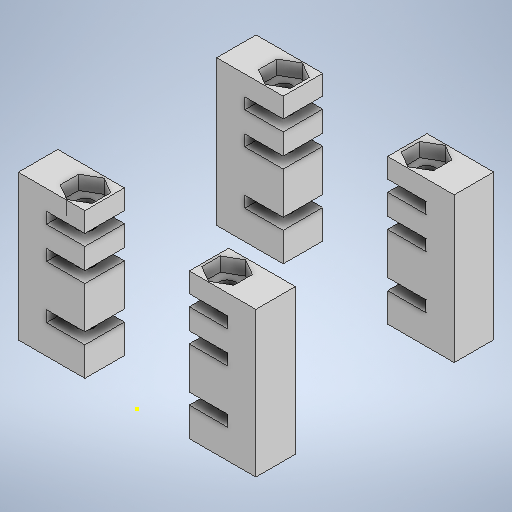
# Autodesk Inventor part: Spacer for PCB boards
Saved by Autodesk Inventor 2025 (Build 290162000, 162)
## iProperties
Created: 2024-07-10
Part Number: Spacer for PCB boards
Material: Generic
Document SubType Name: Modeling
Designer: track
Density: 1 g/cm^3
Appearance: Default
Author: track
## iProperties of the stored document Spacer for PCB boards_3DPrint.ipt
Created: 2024-07-10
Part Number: Spacer for PCB boards_3DPrint
Material: Generic
Document SubType Name: Modeling
Designer: track
Density: 1 g/cm^3
Appearance: Default
Author: track
Autodesk Inventor part; units mm, degrees
ref_plane "YZ Plane" through (0, 0, 0) normal (1, 0, 0) x (0, 1, 0)
ref_plane "XZ Plane" through (0, 0, 0) normal (0, 1, 0) x (-1, 0, 0)
ref_plane "XY Plane" through (0, 0, 0) normal (0, 0, 1) x (1, 0, 0)
sketch "Sketch8" plane through (0, 0, 0) normal (0, 1, 0) x (-1, 0, 0)
  line L0 (-16.05, 21.075) -> (16.05, 21.075)
  line L1 (16.05, 21.075) -> (16.05, -21.075)
  line L2 (16.05, -21.075) -> (-16.05, -21.075)
  line L3 (-16.05, -21.075) -> (-16.05, 21.075)
  line L4 (-16.05, 21.075) -> (16.05, -21.075) construction
  line L5 (16.05, 21.075) -> (-16.05, -21.075) construction
  circle A0 centre (12.65, -17.575) radius 1.5
  line L6 (12.65, -19.075) -> (12.65, -21.075) construction
  line L7 (14.15, -17.575) -> (16.05, -17.575) construction
  line L8 (12.65, -17.575) -> (12.65, -19.075) construction
  line L9 (12.65, -17.575) -> (14.15, -17.575) construction
  line L10 (0, -21.075) -> (0, 21.075) construction
  line L11 (16.05, 0) -> (-16.05, 0) construction
  line L12 (9.25, -14.075) -> (16.05, -14.075)
  line L13 (16.05, -14.075) -> (16.05, -21.075)
  line L14 (16.05, -21.075) -> (9.25, -21.075)
  line L15 (9.25, -21.075) -> (9.25, -14.075)
  line L16 (9.25, -14.075) -> (16.05, -21.075) construction
  line L17 (16.05, -14.075) -> (9.25, -21.075) construction
  circle A1 centre (-12.55, -17.675) radius 1.5
  line L18 (-9.25, -14.075) -> (-16.05, -14.075)
  line L19 (-9.25, -21.075) -> (-9.25, -14.075)
  circle A2 centre (12.55, 17.675) radius 1.5
  line L20 (9.25, 14.075) -> (16.05, 14.075)
  line L21 (9.25, 21.075) -> (9.25, 14.075)
  line L22 (-9.25, 21.075) -> (-9.25, 14.075)
  circle A3 centre (-12.55, 17.475) radius 1.5
  line L23 (-9.25, 14.075) -> (-16.05, 14.075)
  line L24 (16.05, -21.075) -> (22.85, -21.075)
  line L25 (22.85, -21.075) -> (22.85, -14.075)
  line L26 (22.85, -14.075) -> (16.05, -14.075)
  line L27 (16.05, -14.075) -> (16.05, -21.075)
  line L28 (-16.05, -21.075) -> (-22.85, -21.075)
  line L29 (-22.85, -21.075) -> (-22.85, -14.075)
  line L30 (-22.85, -14.075) -> (-16.05, -14.075)
  line L31 (16.05, 21.075) -> (22.85, 21.075)
  line L32 (22.85, 21.075) -> (22.85, 14.075)
  line L33 (22.85, 14.075) -> (16.05, 14.075)
  line L34 (-16.05, 21.075) -> (-22.85, 21.075)
  line L35 (-22.85, 21.075) -> (-22.85, 14.075)
  line L36 (-22.85, 14.075) -> (-16.05, 14.075)
  line L37 (-12.55, -19.175) -> (-12.55, -21.075) construction
  line L38 (-14.05, -17.675) -> (-16.05, -17.675) construction
  line L39 (-14.05, -17.675) -> (-12.55, -17.675) construction
  line L40 (-12.55, -17.675) -> (-12.55, -19.175) construction
  line L41 (-12.55, 17.475) -> (-12.55, 18.975) construction
  line L42 (-12.55, 21.075) -> (-12.55, 18.975) construction
  line L43 (-12.55, 17.475) -> (-14.05, 17.475) construction
  line L44 (-16.05, 17.475) -> (-14.05, 17.475) construction
  line L45 (12.55, 17.675) -> (12.55, 19.175) construction
  line L46 (12.55, 19.175) -> (12.55, 21.075) construction
  line L47 (12.55, 17.675) -> (14.05, 17.675) construction
  line L48 (16.05, 17.675) -> (14.05, 17.675) construction
  point P0 (0, 0)
  dimension "d65" = 42.15
  dimension "d66" = 32.1
  dimension "d67" = 3
  dimension "d69" = 2
  dimension "d70" = 1.9
  dimension "d113" = 3
  dimension "d115" = 1.9
  dimension "d116" = 2
  dimension "d117" = 2
  dimension "d118" = 2.1
  dimension "d119" = 3
  dimension "d120" = 1.9
  dimension "d121" = 2
  dimension "d122" = 3
  constraints: 98 end point, 18 symmetric about line, 11 perpendicular, 10 point on line, 9 point on circle, 8 midpoint, 6 horizontal, 6 parallel, 4 centre point, 3 collinear, 2 equal length, 2 vertical
  measures "d65" distance of L2.end L0.start
  measures "d66" distance of L1.end L2.end
  measures "d67" diameter of A0
  measures "d69" distance of L6.start L6.end
  measures "d70" distance of L7.start L7.end
  measures "d113" diameter of A1
  measures "d115" distance of L37.start L37.end
  measures "d116" distance of L38.start L38.end
  measures "d117" distance of L44.start L43.end
  measures "d118" distance of L42.start L41.end
  measures "d119" diameter of A3
  measures "d120" distance of L45.end L46.end
  measures "d121" distance of L48.start L47.end
  measures "d122" diameter of A2
extrude "Extrusion4" add sketch "Sketch8" along normal blind 1 contours L0 L22 L23 L3 | L3 L36 L35 L34 | L0 L1 L20 L21 | L18 L19 L2 L3 | L3 L28 L29 L30 | L31 L32 L33 L1 | L26 L25 L24 L1 | L1 L2 L15 L12
sketch "Sketch9" plane through (0, 1, 0) normal (0, 1, 0) x (1, 0, 0)
  line L0 (-22.85, 21.075) -> (-22.85, 14.075) projected
  line L1 (-22.85, 21.075) -> (-16.05, 21.075)
  line L2 (-16.05, 21.075) -> (-16.05, 14.075)
  line L3 (-16.05, 14.075) -> (-22.85, 14.075)
  line L4 (-22.85, 14.075) -> (-22.85, 21.075)
  line L5 (-9.25, 21.075) -> (-22.85, 21.075) projected
  line L6 (-16.05, 21.075) -> (-16.05, 14.075) construction
  line L7 (-22.85, 14.075) -> (-9.25, 14.075) projected
  line L8 (0, 20.6342) -> (0, -21.4805) construction
  line L9 (-22.8069, 0) -> (21.3685, 0) construction
  line L10 (22.85, 21.075) -> (22.85, 14.075)
  line L11 (22.85, 21.075) -> (16.05, 21.075)
  line L12 (16.05, 21.075) -> (16.05, 14.075)
  line L13 (16.05, 14.075) -> (22.85, 14.075)
  line L14 (22.85, 14.075) -> (22.85, 21.075)
  line L15 (16.05, 21.075) -> (22.85, 21.075)
  line L16 (22.85, 14.075) -> (16.05, 14.075)
  line L17 (-22.85, -21.075) -> (-22.85, -14.075)
  line L18 (-22.85, -21.075) -> (-16.05, -21.075)
  line L19 (-16.05, -21.075) -> (-16.05, -14.075)
  line L20 (-16.05, -14.075) -> (-22.85, -14.075)
  line L21 (-22.85, -14.075) -> (-22.85, -21.075)
  line L22 (-16.05, -21.075) -> (-22.85, -21.075)
  line L23 (-16.05, -21.075) -> (-16.05, -14.075) construction
  line L24 (-22.85, -14.075) -> (-16.05, -14.075)
  line L25 (0, -20.6342) -> (0, 21.4805) construction
  line L26 (22.85, -21.075) -> (22.85, -14.075)
  line L27 (22.85, -21.075) -> (16.05, -21.075)
  line L28 (16.05, -14.075) -> (22.85, -14.075)
  line L29 (22.85, -14.075) -> (22.85, -21.075)
  line L30 (16.05, -21.075) -> (22.85, -21.075)
  line L31 (22.85, -14.075) -> (16.05, -14.075)
  line L32 (16.05, -21.075) -> (16.05, -14.075)
  point P0 (0, 0)
  point P1 (9.25, 21.075)
  point P2 (9.25, 14.075)
  point P3 (-9.25, -21.075)
  point P4 (-9.25, -14.075)
  point P5 (9.25, -21.075)
  point P6 (9.25, -14.075)
  dimension "d73" = 0
  dimension "d74" = 0
  constraints: 60 end point, 25 symmetric about line, 2 collinear, 2 horizontal, 2 midpoint, 2 parallel, 1 vertical
  measures "d73" distance from line of point (0, 0) L8
  measures "d74" distance from line of point (0, 0) L9
extrude "Extrusion5" add sketch "Sketch9" along normal blind 22.241
sketch "Sketch11" plane through (-16.05, 1, 21.075) normal (1, 0, 0) x (0, 0, -1)
  line L0 (21.075, -1) -> (21.075, 11.5) construction
  line L1 (0, 0) -> (0, 22.241) projected
  line L2 (7, 0) -> (7, 22.241) projected
  line L3 (0, 4.15) -> (7, 4.15)
  line L4 (0, -1) -> (7, -1) projected
  line L5 (0, 6.15) -> (7, 6.15)
  line L6 (7, -1) -> (7, 22.241) projected
  line L7 (0, 3.15) -> (7, 3.15)
  line L8 (0, 7.15) -> (7, 7.15)
  line L9 (0, 12.55) -> (7, 12.55)
  line L10 (0, 13.55) -> (7, 13.55)
  line L11 (0, 15.55) -> (7, 15.55)
  line L12 (0, 0) -> (0, 22.3006)
  line L13 (7, 0) -> (7, 22.3006)
  line L14 (0, 16.55) -> (7, 16.55)
  line L15 (0, 19.25) -> (7, 19.25)
  line L16 (0, 18.25) -> (7, 18.25)
  line L17 (0, 21.25) -> (7, 21.25)
  line L18 (0, 22.25) -> (7, 22.25)
  line L19 (42.15, 0) -> (42.15, 22.241)
  line L20 (35.15, 0) -> (35.15, 22.241)
  line L21 (42.15, 4.15) -> (35.15, 4.15)
  line L22 (42.15, 6.15) -> (35.15, 6.15)
  line L23 (35.15, -1) -> (35.15, 22.241)
  line L24 (42.15, 3.15) -> (35.15, 3.15)
  line L25 (42.15, 7.15) -> (35.15, 7.15)
  line L26 (42.15, 12.55) -> (35.15, 12.55)
  line L27 (42.15, 13.55) -> (35.15, 13.55)
  line L28 (42.15, 15.55) -> (35.15, 15.55)
  line L29 (42.15, 0) -> (42.15, 22.3006)
  line L30 (35.15, 0) -> (35.15, 22.3006)
  line L31 (42.15, 16.55) -> (35.15, 16.55)
  line L32 (42.15, 19.25) -> (35.15, 19.25)
  line L33 (42.15, 18.25) -> (35.15, 18.25)
  line L34 (42.15, 21.25) -> (35.15, 21.25)
  line L35 (42.15, 22.25) -> (35.15, 22.25)
  line L36 (0, 0) -> (7, 0)
  line L37 (35.15, 0) -> (42.15, 0)
  point P0 (7, 15.55)
  point P1 (7, 22.241)
  point P2 (7, 13.55)
  point P3 (7, 7.15)
  point P4 (7, 6.15)
  point P5 (7, 3.15)
  point P6 (42.15, 7.15)
  point P7 (35.15, 7.15)
  point P8 (35.15, 6.15)
  point P9 (0, 15.55)
  point P10 (7, 15.55)
  point P11 (7, 18.25)
  point P12 (0, 18.25)
  point P13 (7, 16.55)
  dimension "d97" = 5.15
  dimension "d98" = 1
  dimension "d99" = 2
  dimension "d100" = 1
  dimension "d101" = 8.4
  dimension "d102" = 1
  dimension "d103" = 2
  dimension "d104" = 1
  dimension "d105" = 2.7
  dimension "d106" = 1
  dimension "d107" = 1
  dimension "d108" = 2
  constraints: 64 end point, 31 symmetric about line, 24 point on line, 11 perpendicular, 2 horizontal, 2 vertical, 1 collinear, 34 other
  measures "d97" distance between parallel lines of L4 L3
  measures "d98" distance between parallel lines of L3 L7
  measures "d99" distance between parallel lines of L3 L5
  measures "d100" distance between parallel lines of L5 L8
  measures "d101" distance between parallel lines of L9 L3
  measures "d102" distance between parallel lines of L9 L10
  measures "d103" distance between parallel lines of L10 L11
  measures "d104" distance between parallel lines of L14 L11
  measures "d105" distance between parallel lines of L15 L14
  measures "d106" distance between parallel lines of L15 L16
  measures "d107" distance between parallel lines of L17 L18
  measures "d108" distance between parallel lines of L15 L17
extrude "Extrusion6" add sketch "Sketch11" along normal up to surface (6.8 mm away) contours L1 L7 L2 L36 | L1 L3 L2 L7 | L1 L8 L2 L5 | L1 L9 L2 L8 | L1 L10 L2 L9 | L1 L14 L2 L11 | L1 L16 L2 L14 | L1 L15 L2 L16 | L1 L12 L18 L13 L2 L17 | L37 L20 L24 L19 | L24 L20 L21 L19 | L22 L20 L25 L19 | L25 L20 L26 L19 | L26 L20 L27 L19 | L28 L20 L31 L19 | L31 L20 L33 L19 | L33 L20 L32 L19 | L34 L20 L30 L35 L29 L19
sketch "Sketch12" plane through (16.05, 1, 14.075) normal (-1, 0, 0) x (0, 0, 1)
  line L0 (7, -1) -> (0, -1) projected
  line L1 (0, -1) -> (0, 4.15) projected
  line L2 (7, 4.15) -> (0, 4.15) projected
  line L3 (7, -1) -> (7, 4.15) projected
  line L4 (7, 13.55) -> (0, 13.55) projected
  line L5 (7, 6.15) -> (7, 13.55) projected
  line L6 (0, 6.15) -> (7, 6.15) projected
  line L7 (0, 13.55) -> (0, 6.15) projected
  line L8 (0, 15.55) -> (7, 15.55) projected
  line L9 (0, 19.25) -> (0, 15.55) projected
  line L10 (7, 19.25) -> (0, 19.25) projected
  line L11 (7, 15.55) -> (7, 19.25) projected
  line L12 (7, 22.25) -> (0, 22.25) projected
  line L13 (7, 21.25) -> (7, 22.25) projected
  line L14 (0, 21.25) -> (7, 21.25) projected
  line L15 (0, 22.25) -> (0, 21.25) projected
  line L16 (-28.15, 21.25) -> (-28.15, 22.25) projected
  line L17 (-35.15, 21.25) -> (-28.15, 21.25) projected
  line L18 (-35.15, 22.25) -> (-35.15, 21.25) projected
  line L19 (-28.15, 22.25) -> (-35.15, 22.25) projected
  line L20 (-35.15, 15.55) -> (-28.15, 15.55) projected
  line L21 (-28.15, 15.55) -> (-28.15, 19.25) projected
  line L22 (-35.15, 15.55) -> (-28.15, 15.55) projected
  line L23 (-35.15, 19.25) -> (-35.15, 15.55) projected
  line L24 (-28.15, 19.25) -> (-35.15, 19.25) projected
  line L25 (-35.15, 6.15) -> (-28.15, 6.15) projected
  line L26 (-35.15, 13.55) -> (-35.15, 6.15) projected
  line L27 (-28.15, 13.55) -> (-35.15, 13.55) projected
  line L28 (-28.15, 6.15) -> (-28.15, 13.55) projected
  line L29 (-28.15, -1) -> (-35.15, -1) projected
  line L30 (-35.15, -1) -> (-35.15, 4.15) projected
  line L31 (-28.15, 4.15) -> (-35.15, 4.15) projected
  line L32 (-28.15, -1) -> (-28.15, 4.15) projected
extrude "Extrusion7" add sketch "Sketch12" along normal up to surface (6.8 mm away)
sketch "Sketch13" plane through (0, 0, 0) normal (0, -1, 0) x (1, 0, 0)
  line L0 (-22.85, -14.075) -> (-16.05, -14.075) projected
  line L1 (-22.85, -14.075) -> (-21.05, -14.075)
  line L2 (-21.05, -14.075) -> (-21.05, -21.075)
  line L3 (-21.05, -21.075) -> (-22.85, -21.075)
  line L4 (-22.85, -21.075) -> (-22.85, -14.075)
  line L5 (0, 0) -> (0, -21.075) construction
  line L6 (0, 0) -> (23.0249, 0) construction
  line L7 (22.85, -14.075) -> (9.25, -14.075)
  line L8 (22.85, -21.075) -> (9.25, -21.075)
  line L9 (22.85, -14.075) -> (21.05, -14.075)
  line L10 (21.05, -14.075) -> (21.05, -21.075)
  line L11 (21.05, -21.075) -> (22.85, -21.075)
  line L12 (22.85, -21.075) -> (22.85, -14.075)
  line L13 (-22.85, 14.075) -> (-9.25, 14.075)
  line L14 (-22.85, 21.075) -> (-9.25, 21.075)
  line L15 (-22.85, 14.075) -> (-21.05, 14.075)
  line L16 (-21.05, 14.075) -> (-21.05, 21.075)
  line L17 (-21.05, 21.075) -> (-22.85, 21.075)
  line L18 (-22.85, 21.075) -> (-22.85, 14.075)
  line L19 (-16.05, 21.075) -> (-16.05, 14.075)
  line L20 (0, 0) -> (0, 21.075) construction
  line L21 (22.85, 14.075) -> (9.25, 14.075)
  line L22 (22.85, 21.075) -> (9.25, 21.075)
  line L23 (22.85, 14.075) -> (21.05, 14.075)
  line L24 (21.05, 14.075) -> (21.05, 21.075)
  line L25 (21.05, 21.075) -> (22.85, 21.075)
  line L26 (22.85, 21.075) -> (22.85, 14.075)
  circle A0 centre (-12.65, -17.575) radius 1.5
  circle A1 centre (-12.65, -17.575) radius 1.5 projected
  line L27 (-16.05, -14.075) -> (-9.25, -14.075) projected
  line L28 (-16.05, -21.075) -> (-16.05, -14.075) projected
  line L29 (-16.05, -14.075) -> (-16.05, -21.075)
  circle A2 centre (-12.55, 17.675) radius 1.5
  circle A3 centre (-12.55, 17.675) radius 1.5 projected
  circle A4 centre (12.65, -17.575) radius 1.5
  circle A5 centre (12.55, 17.675) radius 1.5
  line L30 (-22.85, -14.075) -> (-9.25, -14.075) projected
  line L31 (-9.25, -21.075) -> (-22.85, -21.075) projected
  point P0 (-21.05, 14.075)
  point P1 (21.05, 14.075)
  point P2 (21.05, -14.075)
  dimension "d109" = 5
  dimension "d111" = 3
  constraints: 54 end point, 26 symmetric about line, 4 centre point, 4 concentric, 3 coincident, 3 equal length, 3 point on line, 2 horizontal, 2 midpoint, 1 perpendicular, 1 vertical, 2 other
  measures "d109" distance between parallel lines of L2 L28
  measures "d111" diameter of A2
extrude "Extrusion8" cut sketch "Sketch13" against normal through all contours L0 L2 L3 L4 | L12 L8 L10 L7 | L18 L14 L16 L13 | L21 L24 L22 L26 | A0 | A2 | A4 | A5
sketch "Sketch14" plane through (0, 23.241, 0) normal (0, 1, 0) x (1, 0, 0)
  circle A0 centre (12.55, -17.675) radius 1.5 projected
  line L0 (9.7, -16.0296) -> (12.55, -14.3841)
  line L1 (12.55, -14.3841) -> (15.4, -16.0296)
  line L2 (15.4, -16.0296) -> (15.4, -19.3204)
  line L3 (15.4, -19.3204) -> (12.55, -20.9659)
  line L4 (12.55, -20.9659) -> (9.7, -19.3204)
  line L5 (9.7, -19.3204) -> (9.7, -16.0296)
  line L6 (0, 0) -> (0, 9.6595)
  line L7 (0, 9.6595) -> (0, 0)
  line L8 (0, 0) -> (7.0736, 0)
  circle A1 centre (12.55, -17.675) radius 1.5
  circle A2 centre (12.65, 17.575) radius 1.5 projected
  line L9 (9.8, 19.2204) -> (12.65, 20.8659)
  line L10 (12.65, 20.8659) -> (15.5, 19.2204)
  line L11 (15.5, 19.2204) -> (15.5, 15.9296)
  line L12 (15.5, 15.9296) -> (12.65, 14.2841)
  line L13 (12.65, 14.2841) -> (9.8, 15.9296)
  line L14 (9.8, 15.9296) -> (9.8, 19.2204)
  circle A3 centre (-12.55, -17.675) radius 1.5 projected
  line L15 (-15.4, -16.0296) -> (-12.55, -14.3841)
  line L16 (-12.55, -14.3841) -> (-9.7, -16.0296)
  line L17 (-9.7, -16.0296) -> (-9.7, -19.3204)
  line L18 (-9.7, -19.3204) -> (-12.55, -20.9659)
  line L19 (-12.55, -20.9659) -> (-15.4, -19.3204)
  line L20 (-15.4, -19.3204) -> (-15.4, -16.0296)
  circle A4 centre (-12.65, 17.575) radius 1.5 projected
  line L21 (-15.5, 19.2204) -> (-12.65, 20.8659)
  line L22 (-12.65, 20.8659) -> (-9.8, 19.2204)
  line L23 (-9.8, 19.2204) -> (-9.8, 15.9296)
  line L24 (-9.8, 15.9296) -> (-12.65, 14.2841)
  line L25 (-12.65, 14.2841) -> (-15.5, 15.9296)
  line L26 (-15.5, 15.9296) -> (-15.5, 19.2204)
  line L27 (21.05, -21.075) -> (21.05, -14.075) projected
  line L28 (21.05, -14.075) -> (16.05, -14.075) projected
  line L29 (16.05, -14.075) -> (16.05, -21.075) projected
  line L30 (16.05, -21.075) -> (21.05, -21.075) projected
  circle A5 centre (12.55, -17.675) radius 1.5 projected
  line L31 (16.05, -21.075) -> (9.25, -21.075) projected
  line L32 (16.05, -21.075) -> (16.05, -14.075) projected
  line L33 (16.05, -14.075) -> (9.25, -14.075) projected
  line L34 (9.25, -14.075) -> (9.25, -21.075) projected
  line L35 (21.05, 14.075) -> (21.05, 21.075) projected
  line L36 (21.05, 21.075) -> (16.05, 21.075) projected
  line L37 (16.05, 21.075) -> (16.05, 14.075) projected
  line L38 (16.05, 14.075) -> (21.05, 14.075) projected
  line L39 (9.25, 21.075) -> (9.25, 14.075) projected
  line L40 (16.05, 14.075) -> (9.25, 14.075) projected
  line L41 (16.05, 14.075) -> (16.05, 21.075) projected
  line L42 (16.05, 21.075) -> (9.25, 21.075) projected
  circle A6 centre (12.65, 17.575) radius 1.5 projected
  line L43 (-21.05, 21.075) -> (-21.05, 14.075) projected
  line L44 (-21.05, 14.075) -> (-16.05, 14.075) projected
  line L45 (-16.05, 14.075) -> (-16.05, 21.075) projected
  line L46 (-16.05, 21.075) -> (-21.05, 21.075) projected
  circle A7 centre (-12.65, 17.575) radius 1.5 projected
  line L47 (-16.05, 21.075) -> (-9.25, 21.075) projected
  line L48 (-16.05, 21.075) -> (-16.05, 14.075) projected
  line L49 (-16.05, 14.075) -> (-9.25, 14.075) projected
  line L50 (-9.25, 14.075) -> (-9.25, 21.075) projected
  line L51 (-9.25, -21.075) -> (-9.25, -14.075) projected
  line L52 (-16.05, -14.075) -> (-9.25, -14.075) projected
  line L53 (-16.05, -14.075) -> (-16.05, -21.075) projected
  line L54 (-16.05, -21.075) -> (-9.25, -21.075) projected
  circle A8 centre (-12.55, -17.675) radius 1.5 projected
  line L55 (-21.05, -14.075) -> (-21.05, -21.075) projected
  line L56 (-21.05, -21.075) -> (-16.05, -21.075) projected
  line L57 (-16.05, -21.075) -> (-16.05, -14.075) projected
  line L58 (-16.05, -14.075) -> (-21.05, -14.075) projected
  dimension "d123" = 5.7
  dimension "d124" = 5.7
  dimension "d125" = 5.7
  dimension "d126" = 5.7
  constraints: 54 end point, 5 coincident, 5 vertical, 1 centre point, 1 collinear, 1 concentric, 1 horizontal, 52 other
  measures "d123" distance between parallel lines of L2 L5
  measures "d124" distance between parallel lines of L11 L14
  measures "d125" distance between parallel lines of L17 L20
  measures "d126" distance between parallel lines of L23 L26
extrude "Extrusion9" add sketch "Sketch14" along normal blind 2.5 contours L30 L29 L28 L27 | L31 L34 L33 L29 | L38 L37 L36 L35 | L40 L39 L42 L37 | L46 L45 L44 L43 | L47 L50 L49 L45 | L54 L53 L52 L51 | L56 L55 L58 L53
sketch "Sketch15" plane through (9.25, 22.25, 21.075) normal (0, 0, 1) x (1, 0, 0)
  point P0 (-9.25, -22.25)
body "Solid2"
